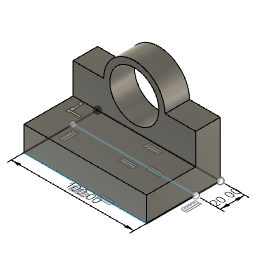
Ex03 (Autodesk Fusion 360 design; units mm, degrees)
Autodesk Fusion 360 part; units mm, degrees
note: some values were not read from the file. Set by a fixed rule: which sketch regions a step uses.
sketch "Sketch1" plane through (0, 0, 0) normal (0, 0, 1) x (1, 0, 0)
  line L0 (0, 0) -> (100, 0)
  line L1 (100, -20) -> (0, -20)
  line L2 (100, 0) -> (100, -60)
  line L3 (100, -60) -> (0, -60)
  line L4 (0, -60) -> (0, 0)
  dimension "d1" = 20
  dimension "d2" = 100
  constraint horizontal L0
  constraint horizontal L1
  constraint coincident L0.start L4.end
  constraint vertical L2
  constraint horizontal L3
  constraint vertical L4
  constraint equal L1 L3
  measures "d1" distance of L0.end L1.start
  measures "d2" distance of L1.start L1.end
extrude "Extrude1" add sketch "Sketch1" along normal blind 45 contours L0 L1 L2 L4
extrude "Extrude2" add sketch "Sketch1" along normal blind 20 contours L1 L2 L3 L4
sketch "Sketch2" plane through (0, -20, 0) normal (0, -1, 0) x (1, 0, 0)
  line L0 (0, 20) -> (100, 20)
  line L1 (100, 20) -> (100, 45)
  line L2 (100, 45) -> (0, 45)
  line L3 (0, 45) -> (0, 20)
  line L4 (50, 10) -> (50, 86.1484) construction
  line L5 (15.2058, 45) -> (84.7942, 45) construction
  circle A0 centre (50, 45) radius 25
  circle A1 centre (50, 45) radius 20
  dimension "d8" = 50
  dimension "d9" = 40
  dimension "d10" = 50
  constraint perpendicular L2 L4
  constraint coincident L2 L5.start
  constraint coincident L2 L5.end
  constraint midpoint L5 A0.centre
  constraint concentric A0 A1
  constraint coincident L4 A0.centre
  measures "d8" diameter of A0
  measures "d9" diameter of A1
  measures "d10" distance of L3 A0.centre
extrude "Extrude3" add sketch "Sketch2" against normal up to surface (20 mm away) contours L2 A0 A1 picked at (26.7597, 46.242)
extrude "Extrude4" cut sketch "Sketch2" against normal up to surface (20 mm away) contours L2 A1 picked at (49.5018, 38.352)
equation "d8 = ( 25 * 2 ) * 1 mm"
